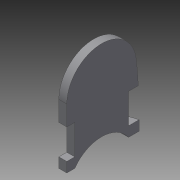
# Autodesk Inventor part: upper_pin
Saved by Autodesk Inventor 2014 (Build 180170000, 170)
## iProperties
Created: 2014-04-25
Part Number: upper_pin
Material: Generic
Document SubType Name: Modeling
Designer: t_emanb
Density: 1 g/cm^3
Appearance: Default
Author: t_emanb
Autodesk Inventor part; units mm, degrees
ref_plane "YZ Plane" through (0, 0, 0) normal (1, 0, 0) x (0, 1, 0)
ref_plane "XZ Plane" through (0, 0, 0) normal (0, 1, 0) x (-1, 0, 0)
ref_plane "XY Plane" through (0, 0, 0) normal (0, 0, 1) x (1, 0, 0)
sketch "Sketch1" plane through (0, 0, 0) normal (1, 0, 0) x (0, 1, 0)
  line L0 (-25.4, -22.225) -> (0, -22.225)
  line L1 (0, -22.225) -> (0, 22.225) construction
  line L2 (0, 22.225) -> (-25.4, 22.225)
  line L3 (-25.4, 22.225) -> (-25.4, -22.225) construction
  line L4 (-25.4, 0) -> (0, 0) construction
  arc A0 (0, -22.225) -> (0, 22.225) centre (0, 0) ccw
  circle A1 centre (-25.4, 0) radius 3.81 construction
  circle A2 centre (0, 0) radius 3.81
  line L5 (-25.4, 22.225) -> (-38.1, 22.225)
  line L6 (-38.1, 22.225) -> (-38.1, -22.225)
  line L7 (-38.1, -22.225) -> (-25.4, -22.225)
  line L8 (0, -5.7) -> (0, 5.7) construction
  line L9 (5.6896, 0) -> (-18.1104, 0) construction
  point P0 (0, 0)
  dimension "d0" = 25.4
  dimension "d1" = 44.45
  dimension "d2" = 7.62
  dimension "d3" = 12.7
  constraints: 20 end point, 4 coincident, 4 parallel, 3 centre point, 2 midpoint, 2 perpendicular, 2 point on circle, 1 collinear, 1 equal radius, 1 horizontal
  measures "d0" distance of L2.end L1.end
  measures "d1" distance of L2.end L0.start
  measures "d2" diameter of A1
  measures "d3" distance between parallel lines of L3 L6
extrude "Extrusion1" add sketch "Sketch1" along normal blind 5.08 contours L7 L6 L5 L2 A0 L0 | A2
sketch "Sketch2" plane through (0, 0, 0) normal (-1, 0, 0) x (0, 0, 1)
  line L0 (-22.225, -38.1) -> (-22.225, 0) projected
  line L1 (22.225, -38.1) -> (-22.225, -38.1) projected
  line L2 (22.225, 0) -> (22.225, -38.1) projected
  line L3 (-22.225, 0) -> (22.225, 0) construction
  line L4 (-22.225, -12.7) -> (-17.145, -12.7)
  line L5 (-17.145, -12.7) -> (-17.145, -31.75)
  line L6 (-17.145, -31.75) -> (-22.225, -31.75)
  line L7 (-22.225, -31.75) -> (-22.225, -12.7)
  line L8 (22.225, -12.7) -> (17.145, -12.7)
  line L9 (17.145, -12.7) -> (17.145, -31.75)
  line L10 (17.145, -31.75) -> (22.225, -31.75)
  line L11 (22.225, -31.75) -> (22.225, -12.7)
  line L12 (0, -38.1) -> (0, 0)
  dimension "d12" = 38.1
  dimension "d13" = 5.08
  dimension "d14" = 5.08
  dimension "d15" = 19.05
  dimension "d16" = 12.7
  constraints: 20 end point, 4 parallel, 4 point on line, 3 perpendicular, 2 collinear, 2 horizontal, 2 midpoint
  measures "d12" distance between parallel lines of L1 L3
  measures "d13" distance of L5.end L6.end
  measures "d14" distance of L9.end L10.end
  measures "d15" distance of L4.end L5.end
  measures "d16" distance between parallel lines of L3 L4
extrude "Extrusion2" cut sketch "Sketch2" against normal through all
sketch "Sketch3" plane through (0, 0, 0) normal (-1, 0, 0) x (0, 0, 1)
  arc A0 (22.225, 0) -> (-22.225, 0) centre (0, 0) ccw projected
  circle A1 centre (0, 0) radius 6.35
  dimension "d19" = 12.7
  constraints: 1 centre point, 1 coincident
  measures "d19" diameter of A1
extrude "Extrusion3" add sketch "Sketch3" along normal blind 2.54
sketch "Sketch4" plane through (-2.54, 0, 0) normal (-1, 0, 0) x (0, 0, 1)
  circle A0 centre (0, 0) radius 6.35 projected
  circle A1 centre (0, 0) radius 3.81
  dimension "d22" = 7.62
  constraints: 1 centre point, 1 coincident
  measures "d22" diameter of A1
extrude "Extrusion4" add sketch "Sketch4" along normal blind 5.08 contours A1
sketch "Sketch5" plane through (-7.62, 0, 0) normal (-1, 0, 0) x (0, 0, 1)
  circle A0 centre (0, 0) radius 3.81 projected
  line L0 (-3.81, 0) -> (3.81, 0)
  constraints: 2 end point, 2 point on circle, 1 horizontal, 1 midpoint
revolve "Revolution1" add sketch "Sketch5" angle 180 about axis through (-7.62, 0, -3.81) along (0, 0, 1) picked at (0.9506, 0.8422) contours L0 A0
sketch "Sketch6" plane through (0, 0, 0) normal (-1, 0, 0) x (0, 0, 1)
  line L0 (-22.225, -38.1) -> (-22.225, -31.75) projected
  line L1 (22.225, -38.1) -> (-22.225, -38.1) projected
  line L2 (-22.225, -12.7) -> (-17.145, -12.7) projected
  line L3 (-17.145, -12.7) -> (-17.145, -31.75) projected
  line L4 (-22.225, -31.75) -> (-23.8687, -31.75)
  spline S0 degree 3 poles (-24.3389, -38.1) (-24.1438, -35.6808) (-23.9932, -34.219) (-23.8687, -31.75) knots -0.835253 -0.835253 -0.835253 -0.835253 -0.05147 -0.05147 -0.05147 -0.05147
  line L5 (-22.225, -38.1) -> (-24.3389, -38.1)
  line L6 (-17.145, -38.1) -> (-17.145, -31.75)
  line L7 (-23.3095, -12.7) -> (-22.225, -12.7)
  line L8 (-17.145, -12.7) -> (-17.145, 0)
  line L9 (-17.145, 0) -> (-22.225, 0)
  spline S1 degree 3 poles (-23.3095, -12.7) (-23.2316, -10.9447) (-23.0986, -8.2586) (-22.7786, -3.8937) (-22.5606, -1.8124) (-22.225, 0) knots -1.036051 -1.036051 -1.036051 -1.036051 -0.552963 -0.552963 0 0 0 0
  line L10 (-22.225, -12.7) -> (-22.225, 0)
  line L11 (-22.225, -31.75) -> (-22.225, -38.1)
  dimension "d26" = 6.35
  dimension "d27" = 6.7237
  dimension "d28" = 7.1939
  dimension "d29" = 12.7
  dimension "d30" = 6.1645
  dimension "d31" = 5.08
  constraints: 16 end point, 5 collinear, 4 horizontal, 3 point on line, 2 vertical, 6 other
  measures "d26" distance of L6.start L6.end
  measures "d27" distance of L6.end L4.end
  measures "d28" distance of L6.start L5.end
  measures "d29" distance of L8.start L8.end
  measures "d30" distance of L7.start L8.start
  measures "d31" distance of L8.end L9.end
extrude "Extrusion5" add sketch "Sketch6" against normal up to surface (5.08 mm away) contours L5 S0 L4 L0 | L7 S1 L10
sketch "Sketch7" plane through (0, -12.7, -17.145) normal (0, -1, 0) x (1, 0, 0)
  line L0 (0, 0) -> (5.08, 0) projected
  line L1 (0, -6.1645) -> (5.08, -6.1645) projected
  line L2 (10.233, 22.3578) -> (10.233, -6.8582) construction
  line L3 (5.08, 0) -> (0, 0)
  line L4 (5.08, -6.1645) -> (5.08, 0)
  spline S0 degree 3 poles (0, -5.08) (1.6825, -5.4909) (3.3765, -5.8525) (5.08, -6.1645) knots -0.570375 -0.570375 -0.570375 -0.570375 -0.050806 -0.050806 -0.050806 -0.050806
  line L5 (0, -5.08) -> (0, 0)
  line L6 (0, 39.37) -> (0, -7.1939) projected
  line L7 (0, -5.08) -> (0, -6.1645)
  line L8 (5.08, -6.1645) -> (0, -6.1645)
  point P0 (0, 17.145)
  dimension "d37" = 5.08
  dimension "d38" = 6.1645
  dimension "d39" = 5.08
  constraints: 12 end point, 4 collinear, 2 vertical, 1 horizontal, 1 point on line, 4 other
  measures "d37" distance of L3.start L3.end
  measures "d38" distance of L4.start L3.start
  measures "d39" distance of L5.start L3.end
extrude "Extrusion6" cut sketch "Sketch7" against normal through all contours S0 L1 L6
sketch "Sketch8" plane through (0, -31.75, -17.145) normal (0, 1, 0) x (1, 0, 0)
  line L0 (0, 0) -> (5.08, 0)
  line L1 (0, 5.08) -> (0, 0)
  spline S0 degree 3 poles (5.08, 6.7237) (3.3633, 6.251) (1.6683, 5.7026) (0, 5.08) knots -0.534217 -0.534217 -0.534217 -0.534217 0 0 0 0
  line L2 (5.08, 0) -> (5.08, 6.7237)
  line L3 (5.08, 6.1645) -> (5.08, 0) projected
  line L4 (0, 0) -> (5.08, 0) projected
  line L5 (5.08, 6.7237) -> (0, 6.7237)
  line L6 (0, 6.7237) -> (0, 5.08)
  line L7 (5.08, 6.7237) -> (5.08, 7.1939) projected
  line L8 (0, 7.1939) -> (5.08, 7.1939) projected
  line L9 (0, 6.7237) -> (0, 7.1939) projected
  line L10 (0, 6.7237) -> (5.08, 6.7237) projected
  line L11 (0, 6.7237) -> (5.08, 6.7237)
  line L12 (5.08, 6.7237) -> (5.08, 7.1939)
  line L13 (5.08, 7.1939) -> (0, 7.1939)
  line L14 (0, 7.1939) -> (0, 6.7237)
  point P0 (0, -17.145)
  dimension "d42" = 5.08
  dimension "d43" = 5.08
  dimension "d44" = 6.7237
  constraints: 18 end point, 2 collinear, 2 horizontal, 2 parallel, 2 vertical, 1 perpendicular, 3 other
  measures "d42" distance of L0.start L0.end
  measures "d43" distance of L1.start L0.start
  measures "d44" distance of L0.end L2.end
extrude "Extrusion7" cut sketch "Sketch8" against normal through all contours L6 L5 S0 | L5 L9 L8 L7
sketch "Sketch9" plane through (0, 0, 0) normal (-1, 0, 0) x (0, 0, 1)
  line L0 (22.225, -38.1) -> (-22.225, -38.1) projected
  line L1 (-17.145, -31.75) -> (-22.225, -31.75) projected
  line L2 (-17.145, -31.75) -> (-17.145, -38.1) construction
  line L3 (17.145, -31.75) -> (17.145, -38.1) construction
  arc A0 (17.145, -38.1) -> (-17.145, -38.1) centre (0, -50.1877) ccw
  line L4 (0, -38.1) -> (0, -29.21) construction
  dimension "d47" = 8.89
  constraints: 6 end point, 3 perpendicular, 3 point on circle, 3 point on line, 1 centre point, 1 midpoint, 1 vertical
  measures "d47" distance of L4.start L4.end
extrude "Extrusion8" cut sketch "Sketch9" against normal through all
fillet "Fillet1" radius 2.54 2 edges at (0, 0, -6.35) (-2.54, 0, -6.35)
body "Solid1"
